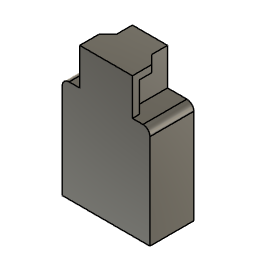
stopper (Autodesk Fusion 360 design; units mm, degrees)
Autodesk Fusion 360 part; units mm, degrees
sketch "Sketch1" plane through (0, 0, 0) normal (0, 0, 1) x (1, 0, 0)
  line L0 (20, 6.5) -> (-20, 6.5)
  line L1 (-20, 6.5) -> (-20, -6.5)
  line L2 (-20, -6.5) -> (20, -6.5)
  line L3 (20, -6.5) -> (20, 6.5)
  line L4 (20, 6.5) -> (-20, -6.5) construction
  line L5 (-20, 6.5) -> (20, -6.5) construction
  dimension "d1" = 40
  dimension "d2" = 13
  constraint horizontal L0
  constraint perpendicular L0 L1
  constraint parallel L0 L2
  constraint parallel L1 L3
  constraint coincident L4 origin
  constraint coincident L5 origin
  measures "d1" distance of L1.end L2.end
  measures "d2" distance of L0.end L1.end
extrude "Extrude1" add sketch "Sketch1" along normal blind 19.5 makes body 1
sketch "Sketch2" plane through (0, 0, 0) normal (0, 0, -1) x (1, 0, 0)
  line L0 (20, -6.5) -> (20, 6.5)
  line L1 (20, 6.5) -> (-20, 6.5)
  line L2 (-20, 6.5) -> (-20, -6.5)
  line L3 (-20, -6.5) -> (20, -6.5)
  circle A0 centre (0, 0) radius 2.15
  dimension "d5" = 4.3
  constraint coincident A0.centre origin
  measures "d5" diameter of A0
extrude "Extrude2" cut sketch "Sketch2" against normal blind 5 contours A0 bodies 1
move_face "OffsetFaces1" offset -12.5 1 faces at (20, -2.1667, 6.5) on bodies 1
move_face "OffsetFaces2" offset -12.5 1 faces at (-20, 2.1667, 6.5) on bodies 1
sketch "Sketch3" plane through (0, 0, 19.5) normal (0, 0, 1) x (-1, 0, 0)
  line L0 (-7.5, 6.5) -> (-7.5, -6.5)
  line L1 (-7.5, -6.5) -> (7.5, -6.5)
  line L2 (7.5, -6.5) -> (7.5, 6.5)
  line L3 (7.5, 6.5) -> (-7.5, 6.5)
  line L4 (-7.5, -6.5) -> (-6, -6.5)
  line L5 (-7.5, -6.5) -> (-7.5, 0)
  line L6 (-6, -6.5) -> (-7.5, 0)
  line L7 (7.5, -6.5) -> (6, -6.5)
  line L8 (7.5, -6.5) -> (7.5, 0)
  line L9 (6, -6.5) -> (7.5, 0)
  dimension "d10" = 1.5
  dimension "d11" = 6.5
  dimension "d12" = 1.5
  dimension "d13" = 6.5
  constraint coincident L0.end L1.start
  constraint perpendicular L0 L4
  constraint perpendicular L1 L5
  constraint coincident L1.end L2.start
  constraint perpendicular L2 L7
  constraint perpendicular L7 L8
  measures "d10" distance of L0.end L4.end
  measures "d11" distance of L0.end L5.end
  measures "d12" distance of L1.end L7.end
  measures "d13" distance of L1.end L8.end
extrude "Extrude3" cut sketch "Sketch3" against normal blind 10 contours L0 L1 L4 L5 L6 | L1 L2 L7 L8 L9 bodies 1
chamfer "Chamfer1" distance 1.4 angle 45 1 edges at (6.75, 3.25, 9.5) on bodies 1
chamfer "Chamfer2" distance 1.4 angle 45 1 edges at (-6.75, 3.25, 9.5) on bodies 1
sketch "Sketch4" plane through (7.5, 0, 0) normal (1, 0, 0) x (0, 1, 0)
  line L0 (0, 10.9) -> (0, 19.5)
  line L1 (0, 19.5) -> (-6.5, 19.5)
  line L2 (-6.5, 19.5) -> (-6.5, 0)
  line L3 (-6.5, 0) -> (6.5, 0)
  line L4 (6.5, 0) -> (6.5, 9.5)
  line L5 (6.5, 9.5) -> (6.2261, 9.5)
  line L6 (6.2261, 9.5) -> (0, 10.9)
  line L7 (6.5, 0) -> (-6.5, 0)
  line L8 (-6.5, 0) -> (-6.5, 9)
  line L9 (-6.5, 9) -> (6.5, 9)
  line L10 (6.5, 9) -> (6.5, 0)
  dimension "d18" = 9
  constraint horizontal L7
  constraint vertical L8
  constraint horizontal L9
  constraint vertical L10
  constraint coincident L3.end L4.start
  measures "d18" distance of L3.end L9.end
extrude "Extrude4" add sketch "Sketch4" along normal blind 5 contours L2 L3 L4 L7 L8 L9 L10 bodies 1
sketch "Sketch5" plane through (-7.5, 0, 0) normal (-1, 0, 0) x (0, -1, 0)
  line L0 (0, 19.5) -> (0, 10.9)
  line L1 (0, 10.9) -> (-6.2261, 9.5)
  line L2 (-6.2261, 9.5) -> (-6.5, 9.5)
  line L3 (-6.5, 9.5) -> (-6.5, 0)
  line L4 (-6.5, 0) -> (6.5, 0)
  line L5 (6.5, 0) -> (6.5, 19.5)
  line L6 (6.5, 19.5) -> (0, 19.5)
  line L7 (6.5, 0) -> (-6.5, 0)
  line L8 (-6.5, 0) -> (-6.5, 9)
  line L9 (-6.5, 9) -> (6.5, 9)
  line L10 (6.5, 9) -> (6.5, 0)
  dimension "d21" = 9
  constraint horizontal L7
  constraint vertical L8
  constraint horizontal L9
  constraint vertical L10
  constraint coincident L4.end L5.start
  measures "d21" distance of L4.end L9.end
extrude "Extrude5" add sketch "Sketch5" along normal blind 5 contours L3 L4 L5 L7 L8 L9 L10 bodies 1
sketch "Sketch6" plane through (0, 0, 19.5) normal (0, 0, 1) x (-1, 0, 0)
  line L0 (6, -6.5) -> (7.5, 0)
  line L1 (7.5, 0) -> (7.5, 6.5)
  line L2 (7.5, 6.5) -> (-7.5, 6.5)
  line L3 (-7.5, 6.5) -> (-7.5, 0)
  line L4 (-7.5, 0) -> (-6, -6.5)
  line L5 (-6, -6.5) -> (6, -6.5)
  line L6 (-5, -6.5) -> (5, -6.5)
  line L7 (5, -6.5) -> (5, 6.5)
  line L8 (5, 6.5) -> (-5, 6.5)
  line L9 (-5, 6.5) -> (-5, -6.5)
  line L10 (-5, -6.5) -> (5, 6.5) construction
  line L11 (5, -6.5) -> (-5, 6.5) construction
  dimension "d24" = 10
  constraint horizontal L6
  constraint perpendicular L6 L7
  constraint parallel L6 L8
  constraint parallel L7 L9
  constraint coincident L10 origin
  constraint coincident L11 origin
  measures "d24" distance of L7.end L8.end
extrude "Extrude6" cut sketch "Sketch6" against normal blind 10.5 contours L0 L1 L2 L5 L7 | L2 L3 L4 L5 L9 bodies 1
sketch "Sketch7" plane through (0, 6.5, 0) normal (0, 1, 0) x (-1, 0, 0)
  line L0 (5, 9) -> (5, 19.5)
  line L1 (5, 19.5) -> (-5, 19.5)
  line L2 (-5, 19.5) -> (-5, 9)
  line L3 (-5, 9) -> (-6, 9)
  line L4 (-6, 9) -> (-6, 10.9)
  line L5 (-6, 10.9) -> (-7.4368, 9.5)
  line L6 (-7.4368, 9.5) -> (-7.5, 9.5)
  line L7 (-7.5, 9.5) -> (-7.5, 9)
  line L8 (-7.5, 9) -> (-12.5, 9)
  line L9 (-12.5, 9) -> (-12.5, 0)
  line L10 (-12.5, 0) -> (12.5, 0)
  line L11 (12.5, 0) -> (12.5, 9)
  line L12 (12.5, 9) -> (7.5, 9)
  line L13 (7.5, 9) -> (7.5, 9.5)
  line L14 (7.5, 9.5) -> (7.4368, 9.5)
  line L15 (7.4368, 9.5) -> (6, 10.9)
  line L16 (6, 10.9) -> (6, 9)
  line L17 (6, 9) -> (5, 9)
  line L18 (12.5, 0) -> (-12.5, 0)
  line L19 (-12.5, 0) -> (-12.5, 9)
  line L20 (-12.5, 9) -> (12.5, 9)
  line L21 (12.5, 9) -> (12.5, 0)
  line L22 (12.5, 9) -> (-12.5767, 9)
  line L23 (-12.5767, 9) -> (-12.5767, 12.8374)
  line L24 (-12.5767, 12.8374) -> (12.5, 12.8374)
  line L25 (12.5, 12.8374) -> (12.5, 9)
  line L26 (5, 9) -> (-5, 9)
  line L27 (-5, 9) -> (-5, 19.5)
  line L28 (-5, 19.5) -> (5, 19.5)
  line L29 (5, 19.5) -> (5, 9)
  constraint horizontal L18
  constraint vertical L19
  constraint horizontal L20
  constraint vertical L21
  constraint coincident L8.end L9.start
  constraint coincident L10.end L11.start
  constraint horizontal L22
  constraint vertical L23
  constraint horizontal L24
  constraint vertical L25
  constraint coincident L11.end L12.start
  constraint horizontal L26
  constraint vertical L27
  constraint horizontal L28
  constraint vertical L29
  constraint coincident L1.end L2.start
  constraint coincident L0.start L17.end
extrude "Extrude7" cut sketch "Sketch7" against normal blind 14 contours L0 L12 L13 L14 L15 L16 L17 L20 L22 L24 L25 L29 | L13 L14 L15 L16 L20 L22 | L2 L3 L4 L5 L6 L7 L8 L20 L22 L23 L24 L27 | L4 L5 L6 L7 L20 L22 bodies 1
sketch "Sketch8" plane through (0, 0, 19.5) normal (0, 0, 1) x (-1, 0, 0)
  line L0 (5, -6.5) -> (5, 6.5)
  line L1 (5, 6.5) -> (-5, 6.5)
  line L2 (-5, 6.5) -> (-5, -6.5)
  line L3 (-5, -6.5) -> (5, -6.5)
  line L4 (5, 6.5) -> (2.7077, -6.5)
  line L5 (5, 6.5) -> (18.2005, 6.5) construction
  line L6 (-5, 6.5) -> (-2.7077, -6.5)
  line L7 (-5, 6.5) -> (8.2005, 6.5) construction
  dimension "d29" = 100
  dimension "d30" = 80
  constraint horizontal L5
  constraint coincident L0.end L1.start
  constraint coincident L3 L4.end
  constraint horizontal L7
  constraint coincident L1.end L2.start
  constraint coincident L3 L6.end
  measures "d29" angle of L4 L5
  measures "d30" angle of L6 L7
extrude "Extrude8" cut sketch "Sketch8" against normal blind 10.5 contours L0 L3 L4 | L2 L3 L6 bodies 1
sketch "Sketch9" plane through (0, 0, 19.5) normal (0, 0, 1) x (-1, 0, 0)
  line L0 (2.7077, -6.5) -> (5, 6.5)
  line L1 (5, 6.5) -> (-5, 6.5)
  line L2 (-5, 6.5) -> (-2.7077, -6.5)
  line L3 (-2.7077, -6.5) -> (2.7077, -6.5)
  line L4 (-7.5, -6.5) -> (7.5, -6.5)
  line L5 (7.5, -6.5) -> (7.5, 6.5)
  line L6 (7.5, 6.5) -> (-7.5, 6.5)
  line L7 (-7.5, 6.5) -> (-7.5, -6.5)
  line L8 (-7.5, -6.5) -> (7.5, 6.5) construction
  line L9 (7.5, -6.5) -> (-7.5, 6.5) construction
  dimension "d33" = 15
  constraint horizontal L4
  constraint perpendicular L4 L5
  constraint parallel L4 L6
  constraint parallel L5 L7
  constraint coincident L8 origin
  constraint coincident L9 origin
  measures "d33" distance of L5.end L6.end
extrude "Extrude9" add sketch "Sketch9" against normal blind 10.5 contours L0 L4 L5 L6 | L2 L4 L6 L7 bodies 1
sketch "Sketch10" plane through (-7.5, 0, 0) normal (-1, 0, 0) x (0, -1, 0)
  line L0 (6.5, 19.5) -> (-6.5, 19.5)
  line L1 (-6.5, 19.5) -> (-6.5, 9)
  line L2 (-6.5, 9) -> (6.5, 9)
  line L3 (6.5, 9) -> (6.5, 19.5)
  line L4 (4.5, 17.5) -> (-4.5, 17.5)
  line L5 (-4.5, 17.5) -> (-4.5, 11)
  line L6 (-4.5, 11) -> (4.5, 11)
  line L7 (4.5, 11) -> (4.5, 17.5)
  line L8 (4.5, 17.5) -> (-4.5, 11) construction
  line L9 (-4.5, 17.5) -> (4.5, 11) construction
  line L10 (-4.5, 11) -> (4.5, 11)
  line L11 (4.5, 11) -> (4.5, 9)
  line L12 (4.5, 9) -> (-4.5, 9)
  line L13 (-4.5, 9) -> (-4.5, 11)
  point P0 (0, 14.25)
  dimension "d36" = 9
  dimension "d37" = 6.5
  constraint horizontal L4
  constraint perpendicular L4 L5
  constraint parallel L4 L6
  constraint parallel L5 L7
  constraint coincident L8 P0
  constraint coincident L9 P0
  constraint horizontal L10
  constraint vertical L11
  constraint horizontal L12
  constraint vertical L13
  constraint coincident L2 L11.end
  measures "d36" distance of L5.end L6.end
  measures "d37" distance of L4.end L5.end
extrude "Extrude10" cut sketch "Sketch10" against normal blind 15 contours L2 L6 L10 L11 L12 L13 | L4 L5 L6 L7 L10 bodies 1
extrude "Extrude11" add sketch "Sketch10" against normal blind 12.5 contours L2 L6 L10 L11 L12 L13 | L4 L5 L6 L7 L10 bodies 1
extrude "Extrude12" cut sketch "Sketch10" against normal blind 2.5 contours L2 L6 L10 L11 L12 L13 | L4 L5 L6 L7 L10 bodies 1
sketch "Sketch11" plane through (0, 4.5, 0) normal (0, -1, 0) x (1, 0, 0)
  line L0 (-7.5, 17.5) -> (-7.5, 9)
  line L1 (-7.5, 9) -> (-5, 9)
  line L2 (-5, 9) -> (-5, 17.5)
  line L3 (-5, 17.5) -> (-7.5, 17.5)
  line L4 (-7.5, 9) -> (-5, 9)
  line L5 (-5, 9) -> (-5, 17.5)
  line L6 (-5, 17.5) -> (-7.5, 17.5)
  line L7 (-7.5, 17.5) -> (-7.5, 9)
  constraint horizontal L4
  constraint vertical L5
  constraint horizontal L6
  constraint vertical L7
  constraint coincident L2.end L3.start
  constraint coincident L0.end L1.start
extrude "Extrude13" cut sketch "Sketch11" against normal blind 4 bodies 1
sketch "Sketch12" plane through (0, 4.5, 0) normal (0, -1, 0) x (1, 0, 0)
  line L0 (5, 17.5) -> (5, 9)
  line L1 (5, 9) -> (7.5, 9)
  line L2 (7.5, 9) -> (7.5, 17.5)
  line L3 (7.5, 17.5) -> (5, 17.5)
  line L4 (7.5, 9) -> (5, 9)
  line L5 (5, 9) -> (5, 17.5)
  line L6 (5, 17.5) -> (7.5, 17.5)
  line L7 (7.5, 17.5) -> (7.5, 9)
  constraint horizontal L4
  constraint vertical L5
  constraint horizontal L6
  constraint vertical L7
  constraint coincident L0.start L3.end
  constraint coincident L1.end L2.start
extrude "Extrude14" cut sketch "Sketch12" against normal blind 6 bodies 1
sketch "Sketch13" plane through (0, 6.5, 0) normal (0, 1, 0) x (-1, 0, 0)
  line L0 (-5, 9) -> (-12.5, 9)
  line L1 (-12.5, 9) -> (-12.5, 0)
  line L2 (-12.5, 0) -> (12.5, 0)
  line L3 (12.5, 0) -> (12.5, 9)
  line L4 (12.5, 9) -> (5, 9)
  line L5 (5, 9) -> (5, 17.5)
  line L6 (5, 17.5) -> (7.5, 17.5)
  line L7 (7.5, 17.5) -> (7.5, 19.5)
  line L8 (7.5, 19.5) -> (-7.5, 19.5)
  line L9 (-7.5, 19.5) -> (-7.5, 17.5)
  line L10 (-7.5, 17.5) -> (-5, 17.5)
  line L11 (-5, 17.5) -> (-5, 9)
  line L12 (7.5, 17.5) -> (5, 17.5)
  line L13 (5, 17.5) -> (5, 19.5)
  line L14 (5, 19.5) -> (7.5, 19.5)
  line L15 (7.5, 19.5) -> (7.5, 17.5)
  line L16 (-7.5, 17.5) -> (-5, 17.5)
  line L17 (-5, 17.5) -> (-5, 19.5)
  line L18 (-5, 19.5) -> (-7.5, 19.5)
  line L19 (-7.5, 19.5) -> (-7.5, 17.5)
  constraint horizontal L12
  constraint vertical L13
  constraint horizontal L14
  constraint vertical L15
  constraint coincident L8 L13.end
  constraint coincident L6.end L7.start
  constraint horizontal L16
  constraint vertical L17
  constraint horizontal L18
  constraint vertical L19
  constraint coincident L8 L17.end
  constraint coincident L9.end L10.start
extrude "Extrude15" cut sketch "Sketch13" against normal blind 5 contours L8 L9 L10 L16 L17 L18 L19 | L6 L7 L8 L12 L13 L14 L15 bodies 1
chamfer "Chamfer3" distance 2.5 angle 45 2 edges at (-7.5, 1.5, 18.5) (7.5, 1.5, 18.5) on bodies 1
move_face "OffsetFaces3" offset -0.5 1 faces at (-1.6667, 6.5, 3) on bodies 1
move_face "OffsetFaces4" offset -0.05 1 faces at (2.1473, 0.1072, 3.3333) on bodies 1
split "Split1" by plane through (0, 0, 9) normal (0, 0, 1) bodies 1 makes body 2 at (1.6667, -3.8333, 19.5)
move_body "Move1" bodies 2 to x (1, 0, 0) y (0, 1, 0) z (0, 0, 1) at (0, 0, 20)
move_face "OffsetFaces5" offset 20 3 faces at (-8.3333, 2.5, 9) (-1.6667, 2.5, 9) (8.3333, 2.5, 9) on bodies 1
combine "Combine1" operation add target body 1 tool bodies 2
fillet "Fillet1" radius 2 2 edges at (12.5, -0.25, 29) (-12.5, -0.25, 29) on bodies 1
